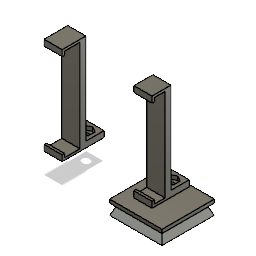
Phone Tripod adapter v1 (Autodesk Fusion 360 design; units mm, degrees)
Autodesk Fusion 360 part; units mm, degrees
sketch "Sketch1" plane through (0, 0, 0) normal (1, 0, 0) x (0, 0, -1)
  line L0 (0, 0) -> (-5, 0)
  line L1 (-5, 0) -> (-5, 75.9)
  line L2 (-5, 75.9) -> (0, 75.9)
  line L3 (0, 75.9) -> (0, 0)
  line L4 (-5, 75.9) -> (-13.7, 75.9)
  line L5 (-13.7, 75.9) -> (-13.7, 77.9)
  line L6 (-13.7, 77.9) -> (-5, 77.9)
  line L7 (-5, 77.9) -> (-5, 75.9)
  line L8 (-5, 77.9) -> (0, 77.9)
  line L9 (0, 77.9) -> (0, 75.9)
  line L10 (0, 75.9) -> (-5, 75.9)
  line L11 (-5, 75.9) -> (-5, 77.9)
  line L12 (-13.7, 77.9) -> (-15.7, 77.9)
  line L13 (-15.7, 77.9) -> (-15.7, 72.9)
  line L14 (-15.7, 72.9) -> (-13.7, 72.9)
  line L15 (-13.7, 72.9) -> (-13.7, 77.9)
  line L16 (0, 0) -> (-15.7, 0)
  line L17 (-15.7, 0) -> (-15.7, -2)
  line L18 (-15.7, -2) -> (0, -2)
  line L19 (0, -2) -> (0, 0)
  line L20 (-15.7, -2) -> (-13.7, -2)
  line L21 (-13.7, -2) -> (-13.7, 3)
  line L22 (-13.7, 3) -> (-15.7, 3)
  line L23 (-15.7, 3) -> (-15.7, -2)
  dimension "d1" = 5
  dimension "d2" = 75.9
  dimension "d3" = 8.7
  dimension "d4" = 2
  dimension "d5" = 2
  dimension "d6" = 5
  dimension "d7" = 2
  dimension "d8" = 5
  constraint horizontal L0
  constraint vertical L1
  constraint horizontal L2
  constraint vertical L3
  constraint coincident L0.start L3.end
  constraint horizontal L4
  constraint vertical L5
  constraint horizontal L6
  constraint vertical L7
  constraint horizontal L8
  constraint vertical L9
  constraint horizontal L10
  constraint vertical L11
  constraint horizontal L12
  constraint vertical L13
  constraint horizontal L14
  constraint vertical L15
  constraint horizontal L16
  constraint vertical L17
  constraint horizontal L18
  constraint vertical L19
  constraint horizontal L20
  constraint vertical L21
  constraint horizontal L22
  constraint vertical L23
  measures "d1" distance of L0.start L0.end
  measures "d2" distance of L0.start L2.end
  measures "d3" distance of L1.end L4.end
  measures "d4" distance of L1.end L6.end
  measures "d5" distance of L5.end L12.end
  measures "d6" distance of L5.end L14.end
  measures "d7" distance of L0.start L18.end
  measures "d8" distance of L17.end L22.end
extrude "Extrude1" add sketch "Sketch1" along normal blind 15 makes body 1
sketch "Sketch2" plane through (0, 0, 0) normal (0, 1, 0) x (1, 0, 0)
  line L0 (0, 0) -> (15, 0)
  line L1 (7.5, 0) -> (7.5, 21.6)
  line L2 (7.5, 21.6) -> (29.1, 21.6)
  line L3 (29.1, 21.6) -> (-14.1, 21.6)
  line L4 (-14.1, 21.6) -> (-14.1, -21.6)
  line L5 (-14.1, -21.6) -> (29.1, -21.6)
  line L6 (29.1, -21.6) -> (29.1, 21.6)
  dimension "d11" = 21.6
  dimension "d12" = 21.6
  dimension "d13" = 43.2
  dimension "d14" = 43.2
  constraint coincident L0.start origin
  constraint horizontal L0
  constraint midpoint L0 L1.start
  constraint perpendicular L0 L1
  constraint perpendicular L1 L2
  constraint horizontal L3
  constraint vertical L4
  constraint horizontal L5
  constraint vertical L6
  measures "d11" distance of L1.start L1.end
  measures "d12" distance of L1.end L2.end
  measures "d13" distance of L2.end L3.end
  measures "d14" distance of L2.end L5.end
extrude "Extrude2" add sketch "Sketch2" along normal blind -5 and the other way blind 10 separate body makes body 2
sketch "Sketch3" plane through (0, -10, 0) normal (0, -1, 0) x (1, 0, 0)
  line L0 (29.1, -21.6) -> (29.1, 21.6)
  line L1 (29.1, 21.6) -> (-14.1, 21.6)
  line L2 (-14.1, 21.6) -> (-14.1, -21.6)
  line L3 (-14.1, -21.6) -> (29.1, -21.6)
  line L4 (-10.45, -17.95) -> (25.45, -17.95)
  line L5 (25.45, -17.95) -> (25.45, 17.95)
  line L6 (25.45, 17.95) -> (-10.45, 17.95)
  line L7 (-10.45, 17.95) -> (-10.45, -17.95)
  dimension "d19" = -3.65
extrude "Extrude3" add sketch "Sketch3" along normal blind 8.7 contours L4 L5 L6 L7 bodies 2
draft "Draft1" angle -22.5 neutral plane through (0, -10, 0) pull (0, -1, 0) 4 faces at (-10.45, -15.8, 5.9833) (1.5167, -15.8, -17.95) (25.45, -15.8, -5.9833) (13.4833, -12.9, 17.95) on bodies 2
extrude "Extrude4" cut 1 faces at (0.3, -5, 7.2) along direction (0, -1, 0) blind 2 on bodies 2 bodies 2
sketch "Sketch4" plane through (0, -2, 0) normal (0, -1, 0) x (1, 0, 0)
  line L0 (0, 15.7) -> (0, 0)
  line L1 (0, 0) -> (15, 0)
  line L2 (15, 0) -> (15, 15.7)
  line L3 (15, 15.7) -> (0, 15.7)
  line L4 (0, 0) -> (15, 0)
  line L5 (15, 0) -> (15, -15)
  line L6 (15, -15) -> (0, -15)
  line L7 (0, -15) -> (0, 0)
  dimension "d26" = 15
  constraint horizontal L4
  constraint vertical L5
  constraint horizontal L6
  constraint vertical L7
  constraint coincident L0.end L1.start
  measures "d26" distance of L0.end L6.end
extrude "Extrude5" add sketch "Sketch4" against normal blind 5 contours L1 L4 L5 L6 L7 bodies 1
sketch "Sketch5" plane through (0, 3, 0) normal (0, 1, 0) x (-1, 0, 0)
  line L0 (-15, -15) -> (0, -15)
  line L1 (0, -15) -> (0, 0)
  line L2 (0, 0) -> (-15, 0)
  line L3 (-15, 0) -> (-15, -15)
  line L4 (-15, -7.5) -> (0, -7.5)
  line L5 (-7.5, -7.5) -> (-12.2, -7.5)
  line L6 (-12.2, -10.2135) -> (-7.5, -12.9271)
  line L7 (-7.5, -12.9271) -> (-2.8, -10.2135)
  line L8 (-2.8, -10.2135) -> (-2.8, -4.7865)
  line L9 (-2.8, -4.7865) -> (-7.5, -2.0729)
  line L10 (-7.5, -2.0729) -> (-12.2, -4.7865)
  line L11 (-12.2, -4.7865) -> (-12.2, -10.2135)
  point P0 (-7.5, -7.5)
  dimension "d29" = 4.7
  constraint midpoint L3 L4.start
  constraint midpoint L1 L4.end
  constraint midpoint L4 P0
  constraint perpendicular L1 L5
  constraint coincident P0 L5.start
  measures "d29" distance of P0 L5.end
extrude "Extrude6" cut sketch "Sketch5" against normal blind 3.25 contours L4 L5 L8 L9 L10 L11 | L4 L5 L6 L7 L8 L11 bodies 1
sketch "Sketch6" plane through (0, -0.25, 0) normal (0, 1, 0) x (-1, 0, 0)
  line L0 (-12.2, -4.7865) -> (-12.2, -10.2135)
  line L1 (-12.2, -10.2135) -> (-7.5, -12.9271)
  line L2 (-7.5, -12.9271) -> (-2.8, -10.2135)
  line L3 (-2.8, -10.2135) -> (-2.8, -4.7865)
  line L4 (-2.8, -4.7865) -> (-7.5, -2.0729)
  line L5 (-7.5, -2.0729) -> (-12.2, -4.7865)
  line L6 (-12.2, -7.5) -> (-2.8, -7.5)
  circle A0 centre (-7.5, -7.5) radius 2.45
  dimension "d32" = 4.9
  constraint midpoint L0 L6.start
  constraint midpoint L3 L6.end
  constraint midpoint L6 A0.centre
  measures "d32" diameter of A0
extrude "Extrude7" cut sketch "Sketch6" against normal blind 18.45 contours L6 A0 | L6 A0 bodies 1 2
sketch "Sketch7" plane through (0, -18.7, 0) normal (0, -1, 0) x (1, 0, 0)
  circle A0 centre (7.5, -7.5) radius 2.45
  line L0 (-14.0537, 21.5537) -> (-14.0537, -21.5537)
  line L1 (-14.0537, -21.5537) -> (29.0537, -21.5537)
  line L2 (29.0537, -21.5537) -> (29.0537, 21.5537)
  line L3 (29.0537, 21.5537) -> (-14.0537, 21.5537)
  circle A1 centre (7.5, -7.5) radius 4.45
  dimension "d35" = 8.9
  constraint concentric A0 A1
  measures "d35" diameter of A1
extrude "Extrude8" cut sketch "Sketch7" against normal blind 7.7 contours A1 bodies 2
chamfer "Chamfer1" distance 2 angle 45 1 edges at (9.7842, -11, -6.614) on bodies 2
copy_body "CopyPasteBodies1" bodies 1 makes body 3
move_body "Move1" bodies 3 to x (1, 0, 0) y (0, 1, 0) z (0, 0, 1) at (-70, 0, 0)
move_face "MoveFace1" by (0, 0, 3.9) 4 faces at (-65, 73.9, 13.7) (-65, 76.2333, 15.7) (-65, 1.3333, 15.7) (-65, 1, 13.7) on bodies 3
equation "d11 = ( 43.2 / 2 ) * 1 mm"
equation "d12 = ( 43.2 / 2 ) * 1 mm"
equation "d13 = 21.600 mm * 2"
equation "d14 = 21.600 mm * 2"
equation "d19 = ( -( 43.2 - 35.9 ) / 2 ) * 1 mm"
equation "d29 = ( 9.4 / 2 ) * 1 mm"
equation "d36 = -11.70 mm + 4 mm"
